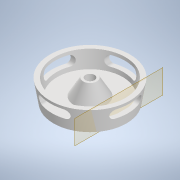
# Autodesk Inventor part: BODY
Saved by Autodesk Inventor 2022 (Build 260153000, 153)
## iProperties
Created: 2022-07-28
Part Number: BODY
Material: Generic
Document SubType Name: Modeling
Designer: Nathan Cai
Density: 1 g/cm^3
Appearance: Default
Author: Nathan Cai
Autodesk Inventor part; units mm, degrees
ref_plane "XZ Plane" through (0, 0, 0) normal (0, 1, 0) x (-1, 0, 0)
ref_plane "XY Plane" through (0, 0, 0) normal (0, 0, 1) x (1, 0, 0)
sketch "Sketch1" plane through (0, 0, 0) normal (0, 0, 1) x (1, 0, 0)
  line L0 (0, 0) -> (17.575, 0)
  line L1 (17.575, 0) -> (17.575, 9.5) construction
  line L2 (17.575, 9.5) -> (0, 9.5)
  line L3 (0, 9.5) -> (0, 0)
  line L4 (17.575, 9.5) -> (16, 0)
  line L5 (15.5477, 9.5) -> (14.3872, 2.5)
  line L6 (14.3872, 2.5) -> (5, 2.5)
  line L7 (5, 0) -> (5, 4)
  line L8 (5, 4) -> (2, 4)
  line L9 (0, 4) -> (2, 4)
  line L10 (2, 4) -> (2, 9.5)
  line L11 (2, 9.5) -> (0, 9.5)
  line L12 (0, 9.5) -> (0, 4)
  line L13 (0, 0) -> (7, 0)
  line L14 (7, 2.5) -> (3, 9.5)
  dimension "d0" = 17.575
  dimension "d1" = 9.5
  dimension "d2" = 16
  dimension "d12" = 2
  dimension "d13" = 2.5
  dimension "d14" = 5
  dimension "d15" = 4
  dimension "d16" = 2
  dimension "d18" = 3
  dimension "d19" = 7
  constraints: 30 end point, 8 point on line, 5 parallel, 3 horizontal, 3 perpendicular
  measures "d0" distance of L2.end L1.end
  measures "d1" distance of L1.end L0.end
  measures "d2" distance from line of L3 L4.end
  measures "d12" distance between parallel lines of L4 L5
  measures "d13" distance between parallel lines of L0 L6
  measures "d14" distance between parallel lines of L3 L7
  measures "d15" distance between parallel lines of L0 L8
  measures "d16" distance of L11.end L10.end
  measures "d18" distance from line of L3 L14.end
  measures "d19" distance from line of L3 L14.start
revolve "Revolution1" add sketch "Sketch1" angle 360 about axis through (0, 9.5, 0) along (0, -1, 0) contours L7 L6 L5 L2 L4 L0 | L7 L8 L10 L2 L14 L6
ref_plane "Work Plane1" through (12.7, 0, 0) normal (1, 0, 0) x (0, 1, 0)
sketch "Sketch2" plane through (12.7, 0, 0) normal (1, 0, 0) x (0, 1, 0)
  line L0 (6.25, 5) -> (6.25, -5) construction
  line L1 (4.25, 5) -> (4.25, -5)
  line L2 (8.25, -5) -> (8.25, 5)
  arc A0 (8.25, 5) -> (4.25, 5) centre (6.25, 5) ccw
  arc A1 (4.25, -5) -> (8.25, -5) centre (6.25, -5) ccw
  line L3 (0, 0) -> (9.5, 0) construction
  line L4 (9.5, 17.575) -> (9.5, -17.575) projected
  line L5 (0, 16) -> (0, -16) projected
  point P0 (6.25, 0)
  dimension "d4" = 5
  dimension "d5" = 4
  dimension "d6" = 4.25
  constraints: 10 end point, 4 point on circle, 4 tangent, 2 centre point, 2 midpoint, 1 parallel, 1 point on line, 1 vertical
  measures "d4" distance of point (6.25, 0) L0.end
  measures "d5" diameter of A1
  measures "d6" distance between parallel lines of L5 L1
extrude "Extrusion1" cut sketch "Sketch2" along normal blind 35.1536
pattern_circular "Circular Pattern1" count 4 over 360 about axis through (0, 4.75, 0) along (0, -1, 0) of "Extrusion1"
body "Solid1"
